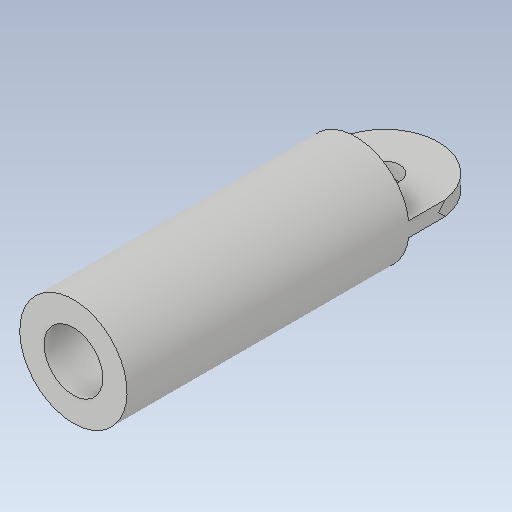
# Autodesk Inventor part: 圓柱
Saved by Autodesk Inventor 2020 (Build 240168000, 168)
## iProperties
Created: 2021-03-25
Part Number: 圓柱
Material: 一般
Document SubType Name: Modeling
Designer: cadlab
Density: 1 g/cm^3
Appearance: 預設
Author: cadlab
Autodesk Inventor part; units mm, degrees
ref_plane "YZ Plane" through (0, 0, 0) normal (1, 0, 0) x (0, 1, 0)
ref_plane "XZ Plane" through (0, 0, 0) normal (0, 1, 0) x (-1, 0, 0)
ref_plane "XY Plane" through (0, 0, 0) normal (0, 0, 1) x (1, 0, 0)
sketch "草圖1" plane through (0, 0, 0) normal (0, 0, 1) x (1, 0, 0)
  circle A0 centre (0, 0) radius 18.272
  dimension "slide_diameter" = 36.544
  constraints: 1 centre point, 1 coincident
  measures "slide_diameter" diameter of A0
extrude "擠出1" add sketch "草圖1" against normal blind 96.127
sketch "草圖2" plane through (0, 0, 0) normal (0, 0, 1) x (1, 0, 0)
  circle A0 centre (0, 0) radius 10
  dimension "hole1" = 20
  constraints: 1 centre point, 1 coincident
  measures "hole1" diameter of A0
extrude "擠出2" cut sketch "草圖2" against normal blind 70
sketch "草圖4" plane through (0, 0, 0) normal (0, 1, 0) x (-1, 0, 0)
  line L0 (18.272, -96.127) -> (18.272, -106.127)
  line L1 (-18.272, -96.127) -> (-18.272, -106.127)
  line L2 (-18.272, -96.127) -> (18.272, -96.127) projected
  line L3 (-18.272, -96.127) -> (18.272, -96.127) projected
  line L4 (-18.272, 0) -> (18.272, 0) projected
  arc A0 (-18.272, -106.127) -> (18.272, -106.127) centre (0, -106.127) ccw
  circle A1 centre (0, -106.127) radius 5
  point P0 (0, 0)
  dimension "center_distance1" = 10
  dimension "hole2" = 10
  constraints: 4 end point, 2 centre point, 2 point on circle, 2 tangent, 1 coincident, 1 parallel, 1 vertical
  measures "center_distance1" distance of L1.start L1.end
  measures "hole2" diameter of A1
extrude "擠出4" add sketch "草圖4" along normal mid plane 5
delete faces "刪除面1" heal yes whole lump no faces at (18.1892, 2.2232, -96.127) (18.1892, -2.2232, -96.127) (-18.1892, 2.2232, -96.127) (-18.1892, -2.2232, -96.127)
